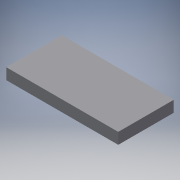
# Autodesk Inventor part: EpoxyFiberMountBase
Saved by Autodesk Inventor 2019 (Build 230136000, 136)
## iProperties
Created: 2019-05-24
Part Number: EpoxyFiberMountBase
Material: Generic
Document SubType Name: Modeling
Designer: aorfi
Density: 1 g/cm^3
Appearance: Default
Author: aorfi
Autodesk Inventor part; units mm, degrees
ref_plane "YZ Plane" through (0, 0, 0) normal (1, 0, 0) x (0, 1, 0)
ref_plane "XZ Plane" through (0, 0, 0) normal (0, 1, 0) x (-1, 0, 0)
ref_plane "XY Plane" through (0, 0, 0) normal (0, 0, 1) x (1, 0, 0)
sketch "Sketch1" plane through (0, 0, 0) normal (0, 1, 0) x (-1, 0, 0)
  line L0 (-10, 4.953) -> (10, 4.953)
  line L1 (10, 4.953) -> (10, -4.953)
  line L2 (10, -4.953) -> (-10, -4.953)
  line L3 (-10, -4.953) -> (-10, 4.953)
  line L4 (-10, 4.953) -> (10, -4.953) construction
  line L5 (10, 4.953) -> (-10, -4.953) construction
  point P0 (0, 0)
  dimension "d0" = 9.906
  dimension "d1" = 20
  constraints: 12 end point, 2 midpoint, 2 parallel, 1 horizontal, 1 perpendicular
  measures "d0" distance of L0.end L1.end
  measures "d1" distance of L0.start L0.end
extrude "Extrusion1" add sketch "Sketch1" along normal mid plane 2
sketch "Sketch2" plane through (-10, -1, 4.953) normal (-1, 0, 0) x (0, 0, 1)
  circle A0 centre (-4.953, 7) radius 1.5875
  circle A1 centre (-4.953, 7) radius 2.75
  line L0 (-7.5076, 8.0181) -> (-9.906, 2)
  line L1 (0, 0) -> (0, 2) projected
  line L2 (-9.906, 2) -> (0, 2)
  line L3 (0, 2) -> (-2.3984, 8.0181)
  point P0 (-4.953, 1)
  dimension "d4" = 3.175
  dimension "d5" = 5.5
  dimension "d6" = 5
  constraints: 6 end point, 2 centre point, 2 point on circle, 2 tangent, 1 coincident, 1 perpendicular, 1 vertical alignment
  measures "d4" diameter of A0
  measures "d5" diameter of A1
  measures "d6" distance from line of L2 A0.centre
extrude "Extrusion2" add sketch "Sketch2" against normal blind 2
mirror "Mirror1" about plane through (0, 0, 0) normal (1, 0, 0) of "Extrusion2"
sketch "Sketch3" plane through (0, 1, 0) normal (0, 1, 0) x (1, 0, 0)
  line L0 (-3.455, 0) -> (3.455, 0) construction
  point P0 (0, 0)
  point P1 (0, 0)
  dimension "d9" = 6.91
  constraints: 2 end point, 1 coincident, 1 horizontal, 1 horizontal alignment, 1 midpoint
  measures "d9" distance of L0.end L0.start
body "Solid1"
